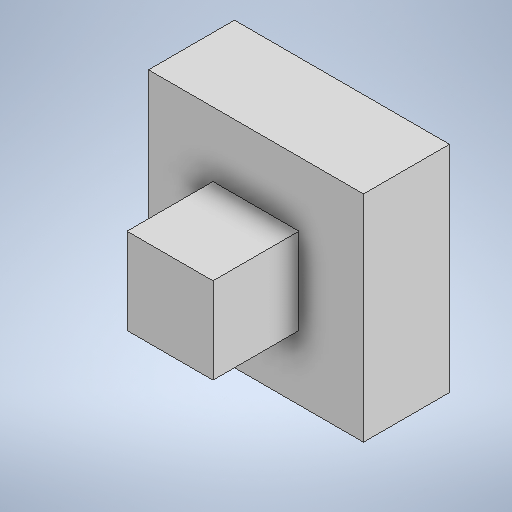
# Autodesk Inventor part: Handle
Saved by Autodesk Inventor 2025.1 (Build 291241020, 241B)
## iProperties
Created: 2024-09-24
Part Number: Handle
Material: Generic
Document SubType Name: Modeling
Designer: jjk
Density: 1 g/cm^3
Appearance: Default
Author: jjk
Autodesk Inventor part; units mm, degrees
ref_plane "YZ Plane" through (0, 0, 0) normal (1, 0, 0) x (0, 1, 0)
ref_plane "XZ Plane" through (0, 0, 0) normal (0, 1, 0) x (-1, 0, 0)
ref_plane "XY Plane" through (0, 0, 0) normal (0, 0, 1) x (1, 0, 0)
sketch "Sketch1" plane through (0, 0, 0) normal (0, 0, 1) x (1, 0, 0)
  line L0 (0, 0) -> (12.7, 0)
  line L1 (12.7, 0) -> (12.7, 12.7)
  line L2 (12.7, 12.7) -> (0, 12.7)
  line L3 (0, 12.7) -> (0, 0)
  dimension "d0" = 12.7
  dimension "d1" = 12.7
  constraints: 8 end point, 2 parallel, 1 horizontal, 1 perpendicular
  measures "d0" distance of L1.end L2.end
  measures "d1" distance of L0.end L1.end
extrude "Extrusion1" add sketch "Sketch1" along normal blind 5.08
sketch "Sketch3" plane through (0, 0, 5.08) normal (0, 0, 1) x (1, 0, 0)
  line L0 (3.81, 8.89) -> (8.89, 8.89)
  line L1 (8.89, 8.89) -> (8.89, 3.81)
  line L2 (8.89, 3.81) -> (3.81, 3.81)
  line L3 (3.81, 3.81) -> (3.81, 8.89)
  line L4 (0, 12.7) -> (0, 0) projected
  line L5 (12.7, 0) -> (12.7, 12.7) projected
  line L6 (12.7, 12.7) -> (0, 12.7) projected
  line L7 (0, 0) -> (12.7, 0) projected
  point P0 (12.7, 6.35)
  dimension "d10" = 3.81
  dimension "d11" = 3.81
  dimension "d12" = 3.81
  dimension "d13" = 3.81
  constraints: 8 end point, 2 parallel, 1 horizontal, 1 midpoint, 1 perpendicular
  measures "d10" distance between parallel lines of L4 L3
  measures "d11" distance from line of point (12.7, 6.35) L1
  measures "d12" distance between parallel lines of L6 L0
  measures "d13" distance between parallel lines of L7 L2
extrude "Extrusion3" add sketch "Sketch3" along normal blind 5.08 contours L0 L1 L2 L3
body "Solid1"
